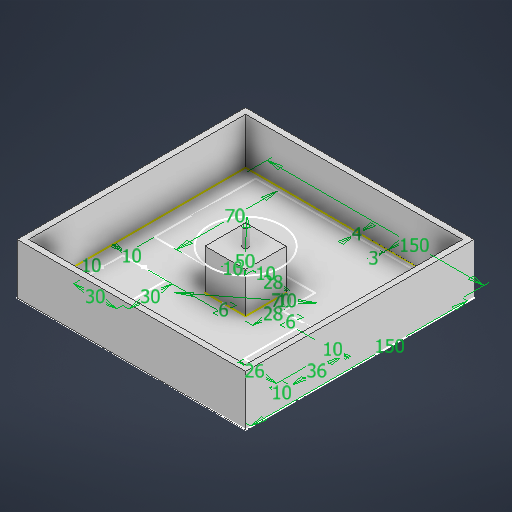
# Autodesk Inventor part: GPS-Compass-casing
Saved by Autodesk Inventor 2026.1 (Build 301233000, 233)
## iProperties
Created: 2025-07-21
Part Number: GPS-Compass-casing
Material: Generic
Document SubType Name: Modeling
Designer: MenMe
Density: 1 g/cm^3
Appearance: Default
Author: MenMe
Autodesk Inventor part; units mm, degrees
ref_plane "YZ Plane" through (0, 0, 0) normal (1, 0, 0) x (0, 1, 0)
ref_plane "XZ Plane" through (0, 0, 0) normal (0, 1, 0) x (-1, 0, 0)
ref_plane "XY Plane" through (0, 0, 0) normal (0, 0, 1) x (1, 0, 0)
sketch "Sketch1" plane through (0, 0, 0) normal (0, 1, 0) x (-1, 0, 0)
  line L0 (-75, 75) -> (75, 75)
  line L1 (75, 75) -> (75, -75)
  line L2 (75, -75) -> (-75, -75)
  line L3 (-75, -75) -> (-75, 75)
  line L4 (-75, 75) -> (75, -75) construction
  line L5 (75, 75) -> (-75, -75) construction
  line L6 (14, 14) -> (-14, 14)
  line L7 (-14, 14) -> (-14, -14)
  line L8 (-14, -14) -> (14, -14)
  line L9 (14, -14) -> (14, 14)
  line L10 (14, 14) -> (-14, -14) construction
  line L11 (-14, 14) -> (14, -14) construction
  circle A0 centre (0, 0) radius 35
  line L12 (-79, -79) -> (79, -79)
  line L13 (79, -79) -> (79, 79)
  line L14 (79, 79) -> (-79, 79)
  line L15 (-79, 79) -> (-79, -79)
  dimension "d0" = 150
  dimension "d1" = 150
  dimension "d2" = 28
  dimension "d3" = 28
  dimension "d4" = 70
  dimension "d7" = 4
  constraints: 32 end point, 6 parallel, 4 midpoint, 3 perpendicular, 2 horizontal, 1 centre point, 1 coincident, 3 other
  measures "d0" distance of L2.end L0.start
  measures "d1" distance of L1.end L2.end
  measures "d2" distance of L8.end L7.end
  measures "d3" distance of L7.end L6.end
  measures "d4" diameter of A0
  measures "d7" distance between parallel lines of L2 L12
extrude "Extrusion2" add sketch "Sketch1" along normal blind 35 contours L15 L14 L13 L12
extrude "Extrusion3" add sketch "Sketch1" along normal blind 3 contours L0 L1 L2 L3 | L9 L8 L7 L6 | A0
sketch "Sketch2" plane through (0, 3, 0) normal (0, 1, 0) x (1, 0, 0)
  line L0 (-14, -14) -> (14, -14)
  line L1 (14, -14) -> (14, 14)
  line L2 (14, 14) -> (-14, 14)
  line L3 (-14, 14) -> (-14, -14)
  line L4 (-14, -14) -> (14, 14) construction
  line L5 (14, -14) -> (-14, 14) construction
  point P0 (0, 0)
  dimension "d12" = 28
  dimension "d13" = 28
  constraints: 12 end point, 2 midpoint, 2 parallel, 1 horizontal, 1 perpendicular
  measures "d12" distance of L2.end L1.end
  measures "d13" distance of L1.end L0.end
extrude "Extrusion4" add sketch "Sketch2" along normal blind 28
sketch "Sketch3" plane through (0, 31, 0) normal (0, 1, 0) x (1, 0, 0)
  circle A0 centre (0, 0) radius 2
  dimension "d16" = 4
  constraints: 1 centre point, 1 coincident
  measures "d16" diameter of A0
extrude "Extrusion5" add sketch "Sketch3" along normal blind 12
sketch "Sketch4" plane through (0, 3, 0) normal (0, 1, 0) x (1, 0, 0)
  line L0 (-65, 72) -> (65, 72)
  line L1 (65, 72) -> (65, 2)
  line L2 (65, 2) -> (24, 2)
  line L3 (24, 2) -> (24, 24)
  line L4 (24, 24) -> (-24, 24)
  line L5 (-24, 24) -> (-24, 2)
  line L6 (-24, 2) -> (-65, 2)
  line L7 (-65, 2) -> (-65, 72)
  line L8 (-75, -75) -> (-75, 75) projected
  line L9 (75, 75) -> (75, -75) projected
  line L10 (-75, 75) -> (75, 75) projected
  line L11 (-14, 14) -> (14, 14) projected
  line L12 (-14, 14) -> (-14, -14) projected
  line L13 (14, 14) -> (14, -14) projected
  line L14 (39, -40) -> (65, -40)
  line L15 (65, -40) -> (65, -4)
  line L16 (65, -4) -> (39, -4)
  line L17 (39, -4) -> (39, -40)
  line L18 (-65, -20) -> (-35, -20)
  line L19 (-35, -20) -> (-35, -50)
  line L20 (-35, -50) -> (-65, -50)
  line L21 (-65, -50) -> (-65, -20)
  line L22 (-14, -14) -> (14, -14) projected
  point P0 (0, 0)
  point P1 (52, -4)
  point P2 (0, -14)
  point P3 (-50, -20)
  point P4 (-65, -35)
  dimension "d19" = 10
  dimension "d20" = 10
  dimension "d21" = 3
  dimension "d22" = 10
  dimension "d23" = 10
  dimension "d24" = 10
  dimension "d25" = 70
  dimension "d26" = 36
  dimension "d29" = 26
  dimension "d30" = 10
  dimension "d31" = 6
  dimension "d33" = 30
  dimension "d34" = 30
  dimension "d36" = 6
  dimension "d37" = 10
  constraints: 32 end point, 7 perpendicular, 4 midpoint, 4 parallel, 2 horizontal, 2 point on line, 1 vertical
  measures "d19" distance between parallel lines of L8 L7
  measures "d20" distance between parallel lines of L9 L1
  measures "d21" distance between parallel lines of L10 L0
  measures "d22" distance between parallel lines of L11 L4
  measures "d23" distance between parallel lines of L12 L5
  measures "d24" distance between parallel lines of L13 L3
  measures "d25" distance between parallel lines of L0 L6
  measures "d26" distance of L15.end L14.end
  measures "d29" distance of L14.start L14.end
  measures "d30" distance between parallel lines of L9 L15
  measures "d31" distance from line of L2 point (52, -4)
  measures "d33" distance of L19.end L20.end
  measures "d34" distance of L18.end L19.end
  measures "d36" distance between parallel lines of L22 L18
  measures "d37" distance from line of L8 point (-65, -35)
sketch "Sketch5" plane through (0, 31, 0) normal (0, 1, 0) x (1, 0, 0)
  circle A0 centre (0, 0) radius 25
  dimension "d32" = 50
  constraints: 1 centre point, 1 coincident
  measures "d32" diameter of A0
body "Solid1"
